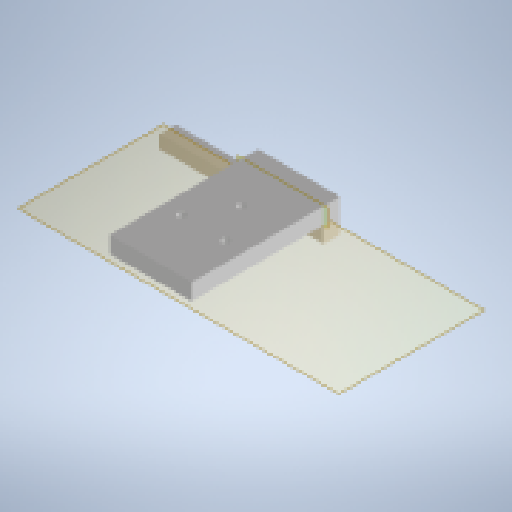
# Autodesk Inventor part: Querplattenaufsatz
Saved by Autodesk Inventor 2024 (Build 280153000, 153)
## iProperties
Created: 2025-09-01
Part Number: Querplattenaufsatz
Material: Generisch
Document SubType Name: Modeling
Designer: weyer
Density: 1 g/cm^3
Appearance: Vorgabe
Author: weyer
Autodesk Inventor part; units mm, degrees
ref_plane "YZ Plane" through (0, 0, 0) normal (1, 0, 0) x (0, 1, 0)
ref_plane "XZ Plane" through (0, 0, 0) normal (0, 1, 0) x (-1, 0, 0)
ref_plane "XY Plane" through (0, 0, 0) normal (0, 0, 1) x (1, 0, 0)
ref_plane "Arbeitsebene1" through (0, 0, 0) normal (0, 0, 1) x (1, 0, 0)
sketch "Skizze1" plane through (0, 0, 0) normal (0, 0, 1) x (1, 0, 0)
  circle A0 centre (-14.875, 15.5) radius 2.45 projected
  circle A1 centre (-28.2984, -7.75) radius 2.45 projected
  circle A2 centre (-1.4516, -7.75) radius 2.45 projected
  line L0 (-72.925, 40.25) -> (85.125, 40.25) projected
  line L1 (85.125, -40.25) -> (-72.925, -40.25) projected
  line L2 (10.125, -40.25) -> (-39.875, -40.25)
  line L3 (-39.875, -40.25) -> (-39.875, 40.25)
  line L4 (-39.875, 40.25) -> (10.125, 40.25)
  line L5 (10.125, 40.25) -> (10.125, -40.25)
  circle A3 centre (-28.2984, -7.75) radius 2.45
  circle A4 centre (-1.4516, -7.75) radius 2.45
  circle A5 centre (-14.875, 15.5) radius 2.45
  point P0 (0, 0)
  dimension "d4" = 25
  dimension "d5" = 50
  constraints: 8 end point, 3 centre point, 3 coincident, 3 concentric, 2 parallel, 2 point on line, 1 horizontal, 1 perpendicular
  measures "d4" distance from line of L3 A0.centre
  measures "d5" distance between parallel lines of L5 L3
extrude "Extrusion1" add sketch "Skizze1" along normal blind 10
ref_plane "Arbeitsebene2" through (-39.875, 40.25, 0) normal (0, 1, 0) x (1, 0, 0)
sketch "Skizze4" plane through (-39.875, 40.25, 0) normal (0, 1, 0) x (1, 0, 0)
  line L0 (50, 0) -> (50, -10) projected
  line L1 (50, -10) -> (50, 18)
  line L2 (50, 18) -> (-48.05, 18)
  line L3 (-48.05, 18) -> (-48.05, 2)
  line L4 (-48.05, 2) -> (8, 2)
  line L5 (8, 2) -> (8, -10)
  line L6 (50, -10) -> (0, -10) projected
  line L7 (50, -10) -> (8, -10)
  line L8 (-48.05, -54) -> (-48.05, 13) projected
  point P0 (39.875, 0)
  dimension "d15" = 28
  dimension "d17" = 90
  dimension "d22" = 0
  dimension "d23" = 98.05
  constraints: 12 end point, 3 perpendicular, 2 vertical, 1 collinear
  measures "d15" distance of L0.end L1.end
  measures "d17" angle of L2 L1
  measures "d22" distance between parallel lines of L3 L8
  measures "d23" distance between parallel lines of L1 L3
extrude "Extrusion3" add sketch "Skizze4" along normal blind 15
